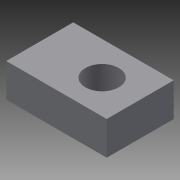
# Autodesk Inventor part: tiedown-hook-clip
Saved by Autodesk Inventor 2015 (Build 190159000, 159)
## iProperties
Created: 2015-02-01
Part Number: tiedown-hook-clip
Material: Generic
Document SubType Name: Modeling
Designer: bovine
Density: 1 g/cm^3
Appearance: Default
Author: bovine
Autodesk Inventor part; units mm, degrees
ref_plane "YZ Plane" through (0, 0, 0) normal (1, 0, 0) x (0, 1, 0)
ref_plane "XZ Plane" through (0, 0, 0) normal (0, 1, 0) x (-1, 0, 0)
ref_plane "XY Plane" through (0, 0, 0) normal (0, 0, 1) x (1, 0, 0)
sketch "Sketch1" plane through (0, 0, 0) normal (0, 1, 0) x (-1, 0, 0)
  line L0 (9.525, 6.35) -> (-9.525, 6.35)
  line L1 (-9.525, 6.35) -> (-9.525, -6.35)
  line L2 (-9.525, -6.35) -> (9.525, -6.35)
  line L3 (9.525, -6.35) -> (9.525, 6.35)
  line L4 (9.525, 6.35) -> (-9.525, -6.35) construction
  line L5 (-9.525, 6.35) -> (9.525, -6.35) construction
  point P0 (0, 0)
  dimension "d0" = 19.05
  dimension "d1" = 12.7
  constraints: 12 end point, 2 midpoint, 2 parallel, 1 horizontal, 1 perpendicular
  measures "d0" distance of L2.end L1.end
  measures "d1" distance of L1.end L0.end
extrude "Extrusion1" add sketch "Sketch1" along normal blind 6.35
sketch "Sketch3" plane through (0, 6.35, 0) normal (0, 1, 0) x (1, 0, 0)
  point P0 (0, 0)
  point P1 (2.2963, 0)
hole "Hole2" at (2.2963, 6.35, 0) direction (0, -1, 0) diameter 6.35 depth 25.4 tip angle 118
body "Solid1"
